Autodesk Fusion 360 part; units mm, degrees
(part 2 of 5)
sketch "Boceto1" plane through (0, 0, 0) normal (0, 1, 0) x (1, 0, 0)
  line L0 (4.8, 0) -> (4.8, -7)
  line L1 (4.8, -7) -> (0, -7)
  line L2 (0, -7) -> (0, 0)
  line L3 (49.6, 0) -> (49.6, -7)
  line L4 (49.6, -7) -> (44.8, -7)
  line L5 (44.8, -7) -> (44.8, 0)
  line L6 (0, 0) -> (-6, 0)
  line L7 (-6, 0) -> (-6, -10)
  line L8 (24.8, 0) -> (24.8, -18)
  line L9 (-2, -14) -> (24.8, -14)
  line L10 (4.8, 0) -> (44.8, 0)
  line L11 (51.6, -14) -> (24.8, -14)
  line L12 (55.6, 0) -> (55.6, -10)
  line L13 (49.6, 0) -> (55.6, 0)
  line L14 (-6, -10) -> (-2, -14)
  line L15 (51.6, -14) -> (55.6, -10)
  line L16 (17.8431, -4) -> (24.8, -11)
  line L17 (17.8431, -4) -> (24.8, -4)
  line L18 (9.8, -3) -> (16.7569, -10)
  line L19 (16.7569, -10) -> (9.8, -10)
  line L20 (9.8, -10) -> (9.8, -3)
  line L21 (39.8, -3) -> (32.8431, -10)
  line L22 (39.8, -10) -> (39.8, -3)
  line L23 (32.8431, -10) -> (39.8, -10)
  line L24 (31.7569, -4) -> (24.8, -4)
  line L25 (31.7569, -4) -> (24.8, -11)
  arc A0 (51.6, -14) -> (-2, -14) centre (24.8, -513.2812) ccw
  point P0 (-6, -14)
  point P1 (55.6, -14)
  dimension "d1" = 4.8
  dimension "d2" = 7
  dimension "d3" = 7
  dimension "d4" = 4.8
  dimension "d5" = 40
  dimension "d6" = 14
  dimension "d8" = 40
  dimension "d9" = 6
  dimension "d10" = 4
  dimension "d11" = 4
  dimension "d12" = 4
  dimension "d13" = 4
  dimension "d14" = 5
  dimension "d15" = 4
  dimension "d16" = 3
  dimension "d17" = 5
  dimension "d18" = 4
  dimension "d19" = 3
  dimension "d26" = 500
  constraint vertical L0
  constraint horizontal L1
  constraint vertical L2
  constraint coincident L2.end L6.start
  constraint vertical L3
  constraint horizontal L4
  constraint vertical L5
  constraint perpendicular L2 L6
  constraint perpendicular L6 L7
  constraint vertical L8
  constraint coincident L8 L9.end
  constraint perpendicular L8 L9
  constraint symmetric L2.end L8 L3.start
  constraint symmetric L6.end L8 L12.start
  constraint symmetric P0 L8 P1
  constraint symmetric L8 L9.end L11.end
  constraint coincident L8.start L10
  constraint coincident L5.end L6
  constraint horizontal L10
  constraint coincident P0 L7
  constraint coincident P0 L9
  constraint coincident P1 L11
  constraint coincident P1 L12
  constraint coincident L8 L16.end
  constraint coincident L8 L17.end
  constraint perpendicular L8 L17
  constraint parallel L17 L19
  constraint vertical L20
  constraint parallel L16 L18
  constraint symmetric L8 L16.start L24.start
  constraint symmetric L8 L16.end L25.end
  constraint symmetric L8 L17.end L24.end
  constraint symmetric L8 L18.start L21.start
  constraint symmetric L8 L18.end L21.end
  constraint symmetric L8 L19.end L22.start
  measures "d1" distance of L2.end L0.start
  measures "d2" distance of L2.end L1.end
  measures "d3" distance of L5.end L4.end
  measures "d4" distance of L5.end L3.start
  measures "d5" distance of L0 L5
  measures "d6" distance of L6.end P0
  measures "d9" distance of L2.end L6.end
  measures "d10" distance of P0 L7.end
  measures "d11" distance of P0 L9.start
  measures "d12" distance of P1 L11.start
  measures "d13" distance of P1 L12.end
  measures "d14" distance of L0 L20
  measures "d15" distance of L9 L19
  measures "d16" distance of L10 L18.start
  measures "d17" distance of L16 L18
  measures "d18" distance of L10 L17
  measures "d19" distance of L11 L16.end
  measures "d26" radius of A0
extrude "Extruir1" add sketch "Boceto1" along normal blind 4.8 contours L0 L1 L2 L6 L7 L8 L10 L14 L16 L17 A0 | L3 L4 L5 L8 L10 L12 L13 L15 L24 L25 A0
fillet "Empalme1" radius 1 9 edges at (9.8, 2.4, 3) (9.8, 2.4, 10) (16.7569, 2.4, 10) (17.8431, 2.4, 4) (24.8, 2.4, 11) (31.7569, 2.4, 4) (32.8431, 2.4, 10) (39.8, 2.4, 3) (39.8, 2.4, 10)
fillet "Empalme2" radius 2.5 4 edges at (-6, 2.4, 10) (55.6, 2.4, 10) (51.6, 2.4, 14) (-2, 2.4, 14)
sketch "Boceto2" plane through (0, 0, 0) normal (0, -1, 0) x (1, 0, 0)
  arc A0 (15.0624, 8.2951) -> (14.3532, 10) centre (14.3532, 9) ccw
  line L0 (15.0624, 8.2951) -> (11.5093, 4.7199)
  arc A1 (9.8, 5.4248) -> (11.5093, 4.7199) centre (10.8, 5.4248) ccw
  line L1 (9.8, 5.4248) -> (9.8, 9)
  arc A2 (10.8, 10) -> (9.8, 9) centre (10.8, 9) ccw
  line L2 (10.8, 10) -> (14.3532, 10)
  arc A3 (39.8, 9) -> (38.8, 10) centre (38.8, 9) ccw
  line L3 (39.8, 9) -> (39.8, 5.4248)
  arc A4 (38.0907, 4.7199) -> (39.8, 5.4248) centre (38.8, 5.4248) ccw
  line L4 (38.0907, 4.7199) -> (34.5376, 8.2951)
  arc A5 (35.2468, 10) -> (34.5376, 8.2951) centre (35.2468, 9) ccw
  line L5 (35.2468, 10) -> (38.8, 10)
  arc A6 (25.5093, 10.2863) -> (24.0907, 10.2863) centre (24.8, 9.5814) ccw
  line L6 (25.5093, 10.2863) -> (30.0624, 5.7049)
  arc A7 (29.3532, 4) -> (30.0624, 5.7049) centre (29.3532, 5) ccw
  line L7 (29.3532, 4) -> (20.2468, 4)
  arc A8 (19.5376, 5.7049) -> (20.2468, 4) centre (20.2468, 5) ccw
  line L8 (19.5376, 5.7049) -> (24.0907, 10.2863)
  arc A9 (-0.891, 13.9417) -> (-2.7872, 13.2128) centre (-1.0195, 11.445) ccw
  line L9 (-2.7872, 13.2128) -> (-5.2678, 10.7322)
  arc A10 (-5.2678, 10.7322) -> (-6, 8.9645) centre (-3.5, 8.9645) ccw
  line L10 (-6, 8.9645) -> (-6, 0)
  line L11 (-6, 0) -> (0, 0)
  line L12 (0, 0) -> (0, 7)
  line L13 (0, 7) -> (4.8, 7)
  line L14 (4.8, 7) -> (4.8, 0)
  line L15 (4.8, 0) -> (44.8, 0)
  line L16 (44.8, 0) -> (44.8, 7)
  line L17 (44.8, 7) -> (49.6, 7)
  line L18 (49.6, 7) -> (49.6, 0)
  line L19 (49.6, 0) -> (55.6, 0)
  line L20 (55.6, 0) -> (55.6, 8.9645)
  arc A11 (55.6, 8.9645) -> (54.8678, 10.7322) centre (53.1, 8.9645) ccw
  line L21 (54.8678, 10.7322) -> (52.3872, 13.2128)
  arc A12 (52.3872, 13.2128) -> (50.491, 13.9417) centre (50.6195, 11.445) ccw
  arc A13 (-0.891, 13.9417) -> (50.491, 13.9417) centre (24.8, 513.2812) ccw
extrude "Extruir2" add 3 faces at (-2, 1.6, 0) (18.1333, 1.6, 0) (51.6, 1.6, 0) along direction (0, 0, -1) blind 2
chamfer "Chaflán1" distance 1 angle 45 4 edges at (0, 2.4, -2) (4.8, 2.4, -2) (44.8, 2.4, -2) (49.6, 2.4, -2)
sketch "Boceto3" plane through (0, 0, 0) normal (0, -1, 0) x (1, 0, 0)
  line L0 (49.6, -1) -> (50.6, -2)
  line L1 (50.6, -2) -> (55.6, -2)
  line L2 (55.6, -2) -> (55.6, 0)
  line L3 (55.6, 0) -> (55.6, 8.9645)
  arc A0 (55.6, 8.9645) -> (54.8678, 10.7322) centre (53.1, 8.9645) ccw
  line L4 (54.8678, 10.7322) -> (52.3872, 13.2128)
  arc A1 (52.3872, 13.2128) -> (50.491, 13.9417) centre (50.6195, 11.445) ccw
  arc A2 (-0.891, 13.9417) -> (50.491, 13.9417) centre (24.8, 513.2812) ccw
  arc A3 (-0.891, 13.9417) -> (-2.7872, 13.2128) centre (-1.0195, 11.445) ccw
  line L5 (-2.7872, 13.2128) -> (-5.2678, 10.7322)
  arc A4 (-5.2678, 10.7322) -> (-6, 8.9645) centre (-3.5, 8.9645) ccw
  line L6 (-6, 8.9645) -> (-6, -2)
  line L7 (-6, -2) -> (-1, -2)
  line L8 (-1, -2) -> (0, -1)
  line L9 (0, -1) -> (0, 7)
  line L10 (0, 7) -> (4.8, 7)
  line L11 (4.8, 7) -> (4.8, -1)
  line L12 (4.8, -1) -> (5.8, -2)
  line L13 (5.8, -2) -> (43.8, -2)
  line L14 (43.8, -2) -> (44.8, -1)
  line L15 (44.8, -1) -> (44.8, 7)
  line L16 (44.8, 7) -> (49.6, 7)
  line L17 (49.6, 7) -> (49.6, -1)
  arc A5 (15.0624, 8.2951) -> (14.3532, 10) centre (14.3532, 9) ccw
  line L18 (15.0624, 8.2951) -> (11.5093, 4.7199)
  arc A6 (9.8, 5.4248) -> (11.5093, 4.7199) centre (10.8, 5.4248) ccw
  line L19 (9.8, 5.4248) -> (9.8, 9)
  arc A7 (10.8, 10) -> (9.8, 9) centre (10.8, 9) ccw
  line L20 (10.8, 10) -> (14.3532, 10)
  arc A8 (39.8, 9) -> (38.8, 10) centre (38.8, 9) ccw
  line L21 (39.8, 9) -> (39.8, 5.4248)
  arc A9 (38.0907, 4.7199) -> (39.8, 5.4248) centre (38.8, 5.4248) ccw
  line L22 (38.0907, 4.7199) -> (34.5376, 8.2951)
  arc A10 (35.2468, 10) -> (34.5376, 8.2951) centre (35.2468, 9) ccw
  line L23 (35.2468, 10) -> (38.8, 10)
  arc A11 (25.5093, 10.2863) -> (24.0907, 10.2863) centre (24.8, 9.5814) ccw
  line L24 (25.5093, 10.2863) -> (30.0624, 5.7049)
  arc A12 (29.3532, 4) -> (30.0624, 5.7049) centre (29.3532, 5) ccw
  line L25 (29.3532, 4) -> (20.2468, 4)
  arc A13 (19.5376, 5.7049) -> (20.2468, 4) centre (20.2468, 5) ccw
  line L26 (19.5376, 5.7049) -> (24.0907, 10.2863)
equation "d3 = d2"
equation "d4 = d1"
equation "d6 = d2 * 2"
equation "d8 = d5"
equation "d11 = d10"
equation "d13 = d12"
equation "d18 = d15"
equation "d19 = d16"

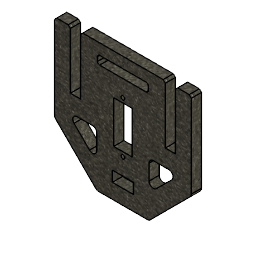
design "SOPORTE SERVO"
Autodesk Fusion 360 part; units mm, degrees
sketch "Boceto1" plane through (0, 0, 0) normal (0, 1, 0) x (1, 0, 0)
  line L0 (0, -1.75) -> (0, -22.5)
  line L1 (-32.3, 1.3953) -> (-32.3, 26)
  line L2 (-32.3, 27.5) -> (47.5, 27.5) construction
  circle A0 centre (0, 27.5) radius 10 construction
  line L3 (-4.35, 39) -> (4.35, 39)
  line L4 (4.35, 39) -> (4.35, 19.1)
  line L5 (4.35, 19.1) -> (-4.35, 19.1)
  line L6 (-4.35, 19.1) -> (-4.35, 39)
  line L7 (-28.6363, 33.7364) -> (-12.7638, 46.7364)
  line L8 (-6.4275, 49) -> (6.4275, 49)
  line L9 (-24.8, -0.2999) -> (-24.8, 27.5)
  line L10 (-24.8, 27.5) -> (-20, 27.5)
  line L11 (-20, 27.5) -> (-20, 0.025)
  line L12 (20, 27.5) -> (20, 0.025)
  line L13 (24.8, -0.2999) -> (24.8, 27.5)
  line L14 (24.8, 27.5) -> (20, 27.5)
  arc A1 (-25.2684, -0.7989) -> (-29.6149, -1.0978) centre (0, -400) ccw
  arc A2 (20, -0.5003) -> (24.8, -0.7695) centre (0, -400) ccw construction
  arc A3 (29.6164, -1.0979) -> (25.2684, -0.7989) centre (0, -400) ccw
  arc A4 (19.4757, -0.4744) -> (-19.4757, -0.4744) centre (0, -400) ccw
  arc A5 (-32.3, 1.3953) -> (-29.6149, -1.0978) centre (-29.8, 1.3953) ccw
  arc A6 (-28.6363, 33.7364) -> (-32.3, 26) centre (-22.3, 26) ccw
  arc A7 (-6.4275, 49) -> (-12.7638, 46.7364) centre (-6.4275, 39) ccw
  arc A8 (29.6149, -1.0978) -> (32.3, 1.3953) centre (29.8, 1.3953) ccw
  line L15 (32.3, 1.3953) -> (32.3, 26)
  arc A9 (32.3, 26) -> (28.6363, 33.7364) centre (22.3, 26) ccw
  line L16 (28.6363, 33.7364) -> (12.7638, 46.7364)
  arc A10 (12.7638, 46.7364) -> (6.4275, 49) centre (6.4275, 39) ccw
  line L17 (20, 27.5) -> (24.8, 27.5)
  circle A11 centre (0, 17) radius 0.9
  line L18 (4.35, 29.05) -> (-4.35, 29.05)
  circle A12 centre (0, 41.1) radius 0.9
  arc A13 (-25.2684, -0.7989) -> (-24.8, -0.2999) centre (-25.3, -0.2999) ccw
  arc A14 (-20, 0.025) -> (-19.4757, -0.4744) centre (-19.5, 0.025) ccw
  arc A15 (19.4757, -0.4744) -> (20, 0.025) centre (19.5, 0.025) ccw
  arc A16 (24.8, -0.2999) -> (25.2684, -0.7989) centre (25.3, -0.2999) ccw
  line L19 (-13, 5) -> (-13, 35.1269)
  line L20 (-11.1681, 38.9951) -> (-11.0225, 39.1144)
  line L21 (-9.39, 38.2925) -> (-11.0012, 4.9517)
  arc A17 (-13, 5) -> (-11.0012, 4.9517) centre (-12, 5) ccw
  arc A18 (-9.39, 38.2925) -> (-11.0225, 39.1144) centre (-10.3889, 38.3407) ccw
  arc A19 (-11.1681, 38.9951) -> (-13, 35.1269) centre (-8, 35.1269) ccw
  arc A20 (13, 35.1269) -> (11.1681, 38.9951) centre (8, 35.1269) ccw
  line L22 (11.1681, 38.9951) -> (11.0225, 39.1144)
  line L23 (9.39, 38.2925) -> (11.0012, 4.9517)
  line L24 (13, 5) -> (13, 35.1269)
  arc A21 (11.0012, 4.9517) -> (13, 5) centre (12, 5) ccw
  arc A22 (11.0225, 39.1144) -> (9.39, 38.2925) centre (10.3889, 38.3407) ccw
  arc A23 (2.8978, 9.7765) -> (0, 6) centre (0, 9) ccw
  line L25 (7.6073, -0.0723) -> (4.8296, 10.2941)
  arc A24 (4.8296, 10.2941) -> (0, 4) centre (0, 9) ccw
  line L26 (2.8978, 9.7765) -> (5.5276, -0.0382)
  arc A25 (0, 4) -> (0, 6) centre (0, 5) ccw
  point P0 (-35.0297, 28.5)
  point P1 (-10, 49)
  point P2 (10, 49)
  point P3 (0, 41.1)
  point P4 (10.3889, 38.3407)
  dimension "d1" = 800
  dimension "d2" = 20
  dimension "d3" = 8.7
  dimension "d4" = 19.9
  dimension "d5" = 4.35
  dimension "d6" = 8.4
  dimension "d7" = 27.5
  dimension "d10" = 20
  dimension "d11" = 10
  dimension "d12" = 10
  dimension "d13" = 4.8
  dimension "d14" = 7.5
  dimension "d15" = 1
  dimension "d17" = 2.5
  dimension "d18" = 10
  dimension "d19" = 1.5
  dimension "d20" = 1.8
  dimension "d21" = 2.1
  dimension "d22" = 0.5
  dimension "d23" = 0.5
  dimension "d24" = 7
  dimension "d25" = 7
  dimension "d30" = 5
  dimension "d32" = 1
  dimension "d33" = 5
  dimension "d36" = 40
  dimension "d37" = 20
  dimension "d38" = 2
  dimension "d39" = 5
  dimension "d41" = 3
  dimension "d42" = 15
  dimension "d43" = 5
  dimension "d44" = 2
  constraint coincident origin A2
  constraint coincident A1.centre L0
  constraint vertical L1
  constraint perpendicular L1 L2
  constraint coincident L0 A0.centre
  constraint horizontal L3
  constraint vertical L4
  constraint horizontal L5
  constraint vertical L6
  constraint coincident L2 A0.centre
  constraint perpendicular L1 L8
  constraint coincident L2 L9.end
  constraint perpendicular L2 L9
  constraint equal A2 A3
  constraint coincident L2 L10.end
  constraint vertical L11
  constraint coincident L1 L2.start
  constraint symmetric L0 L9.end L13.end
  constraint symmetric L0 L10.end L12.start
  constraint concentric A1 A4
  constraint concentric A3 A4
  constraint tangent L1 A5
  constraint tangent A1 A5
  constraint coincident P0 L7
  constraint tangent L1 A6
  constraint tangent L7 A6
  constraint coincident P1 L7
  constraint coincident P1 L8
  constraint tangent L7 A7
  constraint tangent L8 A7
  constraint equal A6 A7
  constraint coincident P2 L8
  constraint symmetric L0 L1.start A8.end
  constraint symmetric L0 A1.end A8.start
  constraint symmetric L0 A5 A8
  constraint symmetric L0 L1.end L15.end
  constraint symmetric L0 L7.start A9.end
  constraint symmetric L0 A6 A9
  constraint symmetric L0 L7.end L16.end
  constraint symmetric L0 L8.start L8.end
  constraint symmetric L0 A7 A10
  constraint coincident A3.start A8
  constraint coincident L0 A11.centre
  constraint midpoint L4 L18.start
  constraint midpoint L6 L18.end
  constraint symmetric A11.centre L18 P3
  constraint symmetric A11 L18 A12
  constraint tangent L9 A13
  constraint tangent A1 A13
  constraint tangent L11 A14
  constraint tangent A4 A14
  constraint equal A13 A14
  constraint coincident A2.start L12
  constraint coincident A2.start A4
  constraint tangent A4 A15
  constraint tangent L12 A15
  constraint equal A13 A15
  constraint coincident A2.end L13
  constraint coincident A2.end A3
  constraint tangent A3 A16
  constraint tangent L13 A16
  constraint equal A1 A2
  constraint equal A2 A4
  constraint vertical L12
  constraint vertical L13
  constraint perpendicular L2 L19
  constraint parallel L7 L20
  constraint tangent L19 A17
  constraint tangent L21 A17
  constraint tangent L21 A18
  constraint tangent L20 A18
  constraint equal A17 A18
  constraint tangent L19 A19
  constraint tangent L20 A19
  constraint symmetric L0 L19.start L24.start
  constraint symmetric L0 L21.end L23.end
  constraint symmetric L0 A17 A21
  constraint symmetric L0 L21.start L23.start
  constraint symmetric L0 L20.end L22.end
  constraint symmetric L0 A18.centre P4
  constraint symmetric L0 L19.end A20.start
  constraint symmetric L0 L20.start A20.end
  constraint symmetric L0 A19 A20
  constraint symmetric L0 A18 A22
  constraint tangent A23 A25
  constraint coincident L0 A25.centre
  constraint coincident L0 A23.centre
  constraint concentric A23 A24
  constraint coincident A2 L25.start
  constraint coincident A2 L26.end
  constraint tangent A23 L26
  constraint parallel L25 L26
  constraint tangent L25 A24
  measures "d1" diameter of A2
  measures "d2" diameter of A0
  measures "d3" distance of L3.start L3.end
  measures "d4" distance of L3.start L5.end
  measures "d5" distance of origin L6
  measures "d6" distance of A0.centre L5
  measures "d7" distance of origin L2
  measures "d10" distance of P1 P2
  measures "d11" distance of L3 L8
  measures "d12" horizontal distance of A0.centre P1
  measures "d13" distance of L9.end L10.end
  measures "d14" distance of L1 L9
  measures "d15" distance of P0 L2
  measures "d17" radius of A5
  measures "d18" radius of A6
  measures "d19" distance of L2 A6.centre
  measures "d20" diameter of A11
  measures "d21" distance of L5 A11.centre
  measures "d22" radius of A13
  measures "d23" radius of A16
  measures "d24" distance of L7 L20
  measures "d25" distance of L11 L19
  measures "d30" distance of L3.start L21
  measures "d32" radius of A17
  measures "d33" radius of A19
  measures "d36" distance of L11 L12
  measures "d37" distance of A0.centre L11
  measures "d38" diameter of A25
  measures "d39" distance of origin A25.centre
  measures "d41" radius of A23
  measures "d42" angle of L0 L26
  measures "d43" vertical distance of origin A17.centre
  measures "d44" distance of A23 A24
extrude "Extruir1" add sketch "Boceto1" along normal blind 4.8 contours L1 L7 L8 L9 L10 L11 L12 L13 L14 A1 A3 A4 A5 A6 A7 A8 L15 A9 L16 A10 L17 A13 A14 A15 A16 A23 L25 A24 L26 A25
sketch "Boceto3" plane through (0, 0, 0) normal (0, -1, 0) x (1, 0, 0)
  arc A0 (9.39, -38.2925) -> (11.0225, -39.1144) centre (10.3889, -38.3407) ccw
  line L0 (9.39, -38.2925) -> (11.0012, -4.9517)
  arc A1 (13, -5) -> (11.0012, -4.9517) centre (12, -5) ccw
  line L1 (13, -5) -> (13, -35.1269)
  arc A2 (11.1681, -38.9951) -> (13, -35.1269) centre (8, -35.1269) ccw
  line L2 (11.1681, -38.9951) -> (11.0225, -39.1144)
  arc A3 (-11.0225, -39.1144) -> (-9.39, -38.2925) centre (-10.3889, -38.3407) ccw
  line L3 (-11.0225, -39.1144) -> (-11.1681, -38.9951)
  arc A4 (-13, -35.1269) -> (-11.1681, -38.9951) centre (-8, -35.1269) ccw
  line L4 (-13, -35.1269) -> (-13, -5)
  arc A5 (-11.0012, -4.9517) -> (-13, -5) centre (-12, -5) ccw
  line L5 (-11.0012, -4.9517) -> (-9.39, -38.2925)
  line L6 (-4.35, -19.1) -> (4.35, -19.1)
  line L7 (4.35, -19.1) -> (4.35, -39)
  line L8 (4.35, -39) -> (-4.35, -39)
  line L9 (-4.35, -39) -> (-4.35, -19.1)
  circle A6 centre (0, -17) radius 0.9
  circle A7 centre (0, -41.1) radius 0.9
  arc A8 (20, -0.025) -> (19.4757, 0.4744) centre (19.5, -0.025) ccw
  arc A9 (7.6073, 0.0723) -> (19.4757, 0.4744) centre (0, 400) ccw
  line L10 (7.6073, 0.0723) -> (4.8296, -10.2941)
  arc A10 (0, -4) -> (4.8296, -10.2941) centre (0, -9) ccw
  arc A11 (0, -6) -> (0, -4) centre (0, -5) ccw
  arc A12 (0, -6) -> (2.8978, -9.7765) centre (0, -9) ccw
  line L11 (2.8978, -9.7765) -> (5.5276, 0.0382)
  arc A13 (-19.4757, 0.4744) -> (5.5276, 0.0382) centre (0, 400) ccw
  arc A14 (-19.4757, 0.4744) -> (-20, -0.025) centre (-19.5, -0.025) ccw
  line L12 (-20, -0.025) -> (-20, -27.5)
  line L13 (-20, -27.5) -> (-24.8, -27.5)
  line L14 (-24.8, -27.5) -> (-24.8, 0.2999)
  arc A15 (-24.8, 0.2999) -> (-25.2684, 0.7989) centre (-25.3, 0.2999) ccw
  arc A16 (-29.6149, 1.0978) -> (-25.2684, 0.7989) centre (0, 400) ccw
  arc A17 (-29.6149, 1.0978) -> (-32.3, -1.3953) centre (-29.8, -1.3953) ccw
  line L15 (-32.3, -1.3953) -> (-32.3, -26)
  arc A18 (-32.3, -26) -> (-28.6363, -33.7364) centre (-22.3, -26) ccw
  line L16 (-28.6363, -33.7364) -> (-12.7638, -46.7364)
  arc A19 (-12.7638, -46.7364) -> (-6.4275, -49) centre (-6.4275, -39) ccw
  line L17 (-6.4275, -49) -> (6.4275, -49)
  arc A20 (6.4275, -49) -> (12.7638, -46.7364) centre (6.4275, -39) ccw
  line L18 (12.7638, -46.7364) -> (28.6363, -33.7364)
  arc A21 (28.6363, -33.7364) -> (32.3, -26) centre (22.3, -26) ccw
  line L19 (32.3, -26) -> (32.3, -1.3953)
  arc A22 (32.3, -1.3953) -> (29.6149, 1.0978) centre (29.8, -1.3953) ccw
  arc A23 (25.2684, 0.7989) -> (29.6149, 1.0978) centre (0, 400) ccw
  arc A24 (25.2684, 0.7989) -> (24.8, 0.2999) centre (25.3, 0.2999) ccw
  line L20 (24.8, 0.2999) -> (24.8, -27.5)
  line L21 (24.8, -27.5) -> (20, -27.5)
  line L22 (20, -27.5) -> (20, -0.025)
  line L23 (-5, -49) -> (5, -49)
  line L24 (5, -49) -> (5, -54)
  line L25 (5, -54) -> (-5, -54)
  line L26 (-5, -54) -> (-5, -49)
  line L27 (-12.3, -61) -> (12.3, -61)
  line L28 (32.3, -41) -> (32.3, -26)
  line L29 (-32.3, -41) -> (-32.3, -26)
  line L30 (12.3, -61) -> (32.3, -41)
  line L31 (-12.3, -61) -> (-32.3, -41)
  arc A25 (-19.4757, 0.4744) -> (19.4757, 0.4744) centre (0, 400) ccw
  line L32 (-20, -0.025) -> (-20, 0.5003)
  line L33 (20, -0.025) -> (20, 0.5003)
  arc A26 (-20, 0.5003) -> (-19.4757, 0.4744) centre (0, 400) ccw
  arc A27 (19.4757, 0.4744) -> (20, 0.5003) centre (0, 400) ccw
  point P0 (-32.3, -61)
  point P1 (32.3, -61)
  dimension "d45" = 5
  dimension "d46" = 5
  dimension "d47" = 10
  dimension "d48" = 7
  dimension "d49" = 20
  dimension "d50" = 20
  dimension "d51" = 20
  dimension "d52" = 20
  constraint horizontal L23
  constraint vertical L24
  constraint horizontal L25
  constraint vertical L26
  constraint coincident L17 L23.start
  constraint perpendicular L26 L27
  constraint coincident A21.end L19.start
  constraint vertical L28
  constraint coincident L15.end A18.start
  constraint vertical L29
  constraint coincident P1 L27
  constraint coincident P1 L28
  constraint coincident P0 L27
  constraint coincident P0 L29
  constraint tangent A9 A25
  constraint tangent A8 A25
  constraint coincident A13.start A14.start
  constraint coincident A14.end L12.start
  constraint vertical L32
  constraint coincident A25 L32.end
  constraint coincident A8.start L22.end
  constraint tangent A8 L33
  constraint equal A25 A26
  constraint coincident A8 A9.end
  constraint coincident A25 L33.end
  constraint coincident L33.end A27.end
  constraint coincident A9.centre A13.centre
  measures "d45" distance of L23.start L25.end
  measures "d46" distance of A7.centre L24
  measures "d47" distance of L24 L26
  measures "d48" distance of L25 L27
  measures "d49" distance of P1 L27.end
  measures "d50" distance of P1 L28.start
  measures "d51" distance of P0 L27.start
  measures "d52" distance of P0 L29.start
extrude "Extruir2" add sketch "Boceto3" against normal blind 4.8 contours A0 L0 A1 L1 A2 L2 | A3 L3 A4 L4 A5 L5 | A8 L33 A27 | L10 A10 A11 A12 L11 A25 | A14 L32 A26 | A18 L16 A19 L17 A20 L18 A21 L24 L25 L26 L27 L28 L29 L30 L31
sketch "Boceto4" plane through (0, 0, 0) normal (0, -1, 0) x (1, 0, 0)
  line L0 (32.3, -41) -> (32.3, -1.3953)
  arc A0 (32.3, -1.3953) -> (29.6149, 1.0978) centre (29.8, -1.3953) ccw
  arc A1 (25.2684, 0.7989) -> (29.6149, 1.0978) centre (0, 400) ccw
  arc A2 (25.2684, 0.7989) -> (24.8, 0.2999) centre (25.3, 0.2999) ccw
  line L1 (24.8, 0.2999) -> (24.8, -27.5)
  line L2 (24.8, -27.5) -> (20, -27.5)
  line L3 (20, -27.5) -> (20, 0.5003)
  arc A3 (-19.4757, 0.4744) -> (20, 0.5003) centre (0, 400) ccw
  line L4 (-20, 0.5003) -> (-20, -27.5)
  line L5 (-20, -27.5) -> (-24.8, -27.5)
  line L6 (-24.8, -27.5) -> (-24.8, 0.2999)
  arc A4 (-24.8, 0.2999) -> (-25.2684, 0.7989) centre (-25.3, 0.2999) ccw
  arc A5 (-29.6149, 1.0978) -> (-25.2684, 0.7989) centre (0, 400) ccw
  arc A6 (-29.6149, 1.0978) -> (-32.3, -1.3953) centre (-29.8, -1.3953) ccw
  line L7 (-32.3, -1.3953) -> (-32.3, -41)
  line L8 (-32.3, -41) -> (-12.3, -61)
  line L9 (-12.3, -61) -> (12.3, -61)
  line L10 (12.3, -61) -> (32.3, -41)
  line L11 (-4.35, -19.1) -> (4.35, -19.1)
  line L12 (4.35, -19.1) -> (4.35, -39)
  line L13 (4.35, -39) -> (-4.35, -39)
  line L14 (-4.35, -39) -> (-4.35, -19.1)
  circle A7 centre (0, -17) radius 0.9
  circle A8 centre (0, -41.1) radius 0.9
  line L15 (5, -49) -> (5, -54)
  line L16 (5, -54) -> (-5, -54)
  line L17 (-5, -54) -> (-5, -49)
  line L18 (-5, -49) -> (5, -49)
  line L19 (-32.3, -7.5) -> (-24.8, -7.5)
  line L20 (24.8, -7.5) -> (32.3, -7.5)
  line L21 (-24.3, -37.6863) -> (-12.35, -49.6363)
  line L22 (-12.35, -49.6363) -> (-12.35, -37.6863)
  line L23 (-24.3, -37.6863) -> (-24.3, -35.5)
  line L24 (-24.3, -35.5) -> (-12.35, -35.5)
  line L25 (-12.35, -35.5) -> (-12.35, -37.6863)
  line L26 (0, 1.75) -> (0, 22.5)
  line L27 (24.3, -37.6863) -> (12.35, -49.6363)
  line L28 (24.3, -37.6863) -> (24.3, -35.5)
  line L29 (24.3, -35.5) -> (12.35, -35.5)
  line L30 (12.35, -49.6363) -> (12.35, -37.6863)
  line L31 (12.35, -35.5) -> (12.35, -37.6863)
  arc A9 (-20, 0.5003) -> (-19.4757, 0.4744) centre (0, 400) ccw
  dimension "d55" = 20
  dimension "d56" = 8
  dimension "d57" = 8
  dimension "d58" = 8
  dimension "d59" = 8
  constraint coincident L7 L19.start
  constraint coincident L6 L19.end
  constraint perpendicular L6 L19
  constraint coincident L1 L20.start
  constraint coincident L0 L20.end
  constraint perpendicular L0 L20
  constraint coincident L19 L20.start
  constraint vertical L22
  constraint parallel L8 L21
  constraint perpendicular L23 L24
  constraint vertical L25
  constraint symmetric L21.start L26 L27.start
  constraint symmetric L21.end L26 L27.end
  constraint symmetric L22.end L26 L30.end
  constraint symmetric L23.end L26 L28.end
  constraint symmetric L24.end L26 L29.end
  measures "d55" distance of L5 L19
  measures "d56" distance of L7 L21.start
  measures "d57" distance of L8 L21
  measures "d58" distance of L14 L22
  measures "d59" distance of L5 L24
extrude "Extruir3" cut sketch "Boceto4" against normal blind 4.8 contours L21 L22 L23 L24 L25 | L27 L28 L29 L30 L31
sketch "Boceto5" plane through (0, 0, 0) normal (0, -1, 0) x (1, 0, 0)
  line L0 (-32.3, -1.3953) -> (-32.3, -41)
  line L1 (-32.3, -41) -> (-12.3, -61)
  line L2 (-12.3, -61) -> (12.3, -61)
  line L3 (12.3, -61) -> (32.3, -41)
  line L4 (32.3, -41) -> (32.3, -1.3953)
  line L5 (24.8, 0.2999) -> (24.8, -27.5)
  line L6 (24.8, -27.5) -> (20, -27.5)
  line L7 (20, -27.5) -> (20, 0.5003)
  arc A0 (-19.4757, 0.4744) -> (20, 0.5003) centre (0, 400) ccw
  line L8 (-20, 0.5003) -> (-20, -27.5)
  line L9 (-20, -27.5) -> (-24.8, -27.5)
  line L10 (-24.8, -27.5) -> (-24.8, 0.2999)
  line L11 (5, -49) -> (5, -54)
  line L12 (5, -54) -> (-5, -54)
  line L13 (-5, -54) -> (-5, -49)
  line L14 (-5, -49) -> (5, -49)
  circle A1 centre (0, -41.1) radius 0.9
  circle A2 centre (0, -17) radius 0.9
  line L15 (-4.35, -19.1) -> (4.35, -19.1)
  line L16 (4.35, -19.1) -> (4.35, -39)
  line L17 (4.35, -39) -> (-4.35, -39)
  line L18 (-4.35, -39) -> (-4.35, -19.1)
  line L19 (12.35, -35.5) -> (24.3, -35.5)
  line L20 (24.3, -35.5) -> (24.3, -37.6863)
  line L21 (24.3, -37.6863) -> (12.35, -49.6363)
  line L22 (12.35, -49.6363) -> (12.35, -35.5)
  line L23 (-12.35, -35.5) -> (-12.35, -49.6363)
  line L24 (-12.35, -49.6363) -> (-24.3, -37.6863)
  line L25 (-24.3, -37.6863) -> (-24.3, -35.5)
  line L26 (-24.3, -35.5) -> (-12.35, -35.5)
  line L27 (-12, -9.1) -> (12, -9.1)
  line L28 (12, -9.1) -> (12, -5.1)
  line L29 (12, -5.1) -> (-12, -5.1)
  line L30 (-12, -5.1) -> (-12, -9.1)
  arc A3 (-24.8, 0.2999) -> (-25.2684, 0.7989) centre (-25.3, 0.2999) ccw
  arc A4 (-29.6149, 1.0978) -> (-25.2684, 0.7989) centre (0, 400) ccw
  arc A5 (-29.6149, 1.0978) -> (-32.3, -1.3953) centre (-29.8, -1.3953) ccw
  arc A6 (32.3, -1.3953) -> (29.6149, 1.0978) centre (29.8, -1.3953) ccw
  arc A7 (25.2684, 0.7989) -> (29.6149, 1.0978) centre (0, 400) ccw
  arc A8 (25.2684, 0.7989) -> (24.8, 0.2999) centre (25.3, 0.2999) ccw
  arc A9 (-20, 0.5003) -> (-19.4757, 0.4744) centre (0, 400) ccw
  dimension "d64" = 10
  dimension "d65" = 8
  dimension "d66" = 8
  dimension "d67" = 4
  constraint horizontal L27
  constraint vertical L28
  constraint horizontal L29
  constraint vertical L30
  measures "d64" distance of L15 L27
  measures "d65" distance of L8 L30
  measures "d66" distance of L7 L28
  measures "d67" distance of L27.end L28.end
extrude "Extruir4" cut sketch "Boceto5" against normal blind 4.8 contours L27 L28 L29 L30
fillet "Empalme2" radius 1 4 edges at (12, 2.4, -5.1) (12, 2.4, -9.1) (-12, 2.4, -9.1) (-12, 2.4, -5.1)
sketch "Boceto6" plane through (0, 0, 0) normal (0, -1, 0) x (1, 0, 0)
  line L0 (11, -9.1) -> (-11, -9.1)
  arc A0 (-12, -8.1) -> (-11, -9.1) centre (-11, -8.1) ccw
  line L1 (-12, -8.1) -> (-12, -6.1)
  arc A1 (-11, -5.1) -> (-12, -6.1) centre (-11, -6.1) ccw
  line L2 (-11, -5.1) -> (11, -5.1)
  arc A2 (12, -6.1) -> (11, -5.1) centre (11, -6.1) ccw
  line L3 (12, -6.1) -> (12, -8.1)
  arc A3 (11, -9.1) -> (12, -8.1) centre (11, -8.1) ccw
  line L4 (-12.35, -35.5) -> (-12.35, -49.6363)
  line L5 (-12.35, -49.6363) -> (-24.3, -37.6863)
  line L6 (-24.3, -37.6863) -> (-24.3, -35.5)
  line L7 (-24.3, -35.5) -> (-12.35, -35.5)
  line L8 (12.35, -35.5) -> (24.3, -35.5)
  line L9 (24.3, -35.5) -> (24.3, -37.6863)
  line L10 (24.3, -37.6863) -> (12.35, -49.6363)
  line L11 (12.35, -49.6363) -> (12.35, -35.5)
  line L12 (32.3, -41) -> (32.3, -1.3953)
  arc A4 (32.3, -1.3953) -> (29.6149, 1.0978) centre (29.8, -1.3953) ccw
  arc A5 (25.2684, 0.7989) -> (29.6149, 1.0978) centre (0, 400) ccw
  arc A6 (25.2684, 0.7989) -> (24.8, 0.2999) centre (25.3, 0.2999) ccw
  line L13 (24.8, 0.2999) -> (24.8, -27.5)
  line L14 (24.8, -27.5) -> (20, -27.5)
  line L15 (20, -27.5) -> (20, 0.5003)
  arc A7 (-19.4757, 0.4744) -> (20, 0.5003) centre (0, 400) ccw
  line L16 (-20, 0.5003) -> (-20, -27.5)
  line L17 (-20, -27.5) -> (-24.8, -27.5)
  line L18 (-24.8, -27.5) -> (-24.8, 0.2999)
  arc A8 (-24.8, 0.2999) -> (-25.2684, 0.7989) centre (-25.3, 0.2999) ccw
  arc A9 (-29.6149, 1.0978) -> (-25.2684, 0.7989) centre (0, 400) ccw
  arc A10 (-29.6149, 1.0978) -> (-32.3, -1.3953) centre (-29.8, -1.3953) ccw
  line L19 (-32.3, -1.3953) -> (-32.3, -41)
  line L20 (-32.3, -41) -> (-12.3, -61)
  line L21 (-12.3, -61) -> (12.3, -61)
  line L22 (12.3, -61) -> (32.3, -41)
  line L23 (-4.35, -19.1) -> (4.35, -19.1)
  line L24 (4.35, -19.1) -> (4.35, -39)
  line L25 (4.35, -39) -> (-4.35, -39)
  line L26 (-4.35, -39) -> (-4.35, -19.1)
  circle A11 centre (0, -17) radius 0.9
  circle A12 centre (0, -41.1) radius 0.9
  line L27 (5, -49) -> (5, -54)
  line L28 (5, -54) -> (-5, -54)
  line L29 (-5, -54) -> (-5, -49)
  line L30 (-5, -49) -> (5, -49)
  line L31 (-32.3, -10.188) -> (-32.3, 0)
  line L32 (-32.3, 0) -> (32.3, 0)
  line L33 (32.3, 0) -> (32.3, -10.3093)
  arc A13 (-20, 0.5003) -> (-19.4757, 0.4744) centre (0, 400) ccw
  dimension "d74" = 27.5
  constraint coincident L19 L31.start
  constraint perpendicular L31 L32
  constraint coincident L12 L33.end
  constraint horizontal L32
  constraint vertical L33
  measures "d74" distance of L14 L32
extrude "Extruir5" cut sketch "Boceto6" against normal blind 4.8 contours A4 A5 A6 L13 L32 | L15 A7 L32 | A7 L16 L32 A13 | L18 A8 A9 A10 L32
extrude "Extruir6" add sketch "Boceto6" against normal blind 4.8 contours A4 L32 L33 | A10 L31 L32
chamfer "Chaflán1" distance 1 angle 45 6 edges at (-32.3, 2.4, 0) (-24.8, 2.4, 0) (-20, 2.4, 0) (20, 2.4, 0) (24.8, 2.4, 0) (32.3, 2.4, 0)
fillet "Empalme4" radius 2 12 edges at (-32.3, 2.4, -41) (-12.35, 2.4, -35.5) (-24.3, 2.4, -35.5) (-24.3, 2.4, -37.6863) (-12.35, 2.4, -49.6363) (-12.3, 2.4, -61) (12.3, 2.4, -61) (12.35, 2.4, -49.6363) (12.35, 2.4, -35.5) (24.3, 2.4, -35.5) (24.3, 2.4, -37.6863) (32.3, 2.4, -41)
sketch "Boceto7" plane through (0, 0, 0) normal (0, -1, 0) x (1, 0, 0)
  line L0 (5, -49) -> (5, -54)
  line L1 (5, -54) -> (-5, -54)
  line L2 (-5, -54) -> (-5, -49)
  line L3 (-5, -49) -> (5, -49)
  circle A0 centre (0, -41.1) radius 0.9
  circle A1 centre (0, -17) radius 0.9
  line L4 (-4.35, -19.1) -> (4.35, -19.1)
  line L5 (4.35, -19.1) -> (4.35, -39)
  line L6 (4.35, -39) -> (-4.35, -39)
  line L7 (-4.35, -39) -> (-4.35, -19.1)
  line L8 (14.35, -35.5) -> (21.6579, -35.5)
  arc A2 (23.0721, -38.9142) -> (21.6579, -35.5) centre (21.6579, -37.5) ccw
  line L9 (23.0721, -38.9142) -> (15.7642, -46.2221)
  arc A3 (12.35, -44.8079) -> (15.7642, -46.2221) centre (14.35, -44.8079) ccw
  line L10 (12.35, -44.8079) -> (12.35, -37.5)
  arc A4 (14.35, -35.5) -> (12.35, -37.5) centre (14.35, -37.5) ccw
  arc A5 (-21.6579, -35.5) -> (-23.0721, -38.9142) centre (-21.6579, -37.5) ccw
  line L11 (-21.6579, -35.5) -> (-14.35, -35.5)
  arc A6 (-12.35, -37.5) -> (-14.35, -35.5) centre (-14.35, -37.5) ccw
  line L12 (-12.35, -37.5) -> (-12.35, -44.8079)
  arc A7 (-15.7642, -46.2221) -> (-12.35, -44.8079) centre (-14.35, -44.8079) ccw
  line L13 (-15.7642, -46.2221) -> (-23.0721, -38.9142)
  line L14 (11, -9.1) -> (-11, -9.1)
  arc A8 (-12, -8.1) -> (-11, -9.1) centre (-11, -8.1) ccw
  line L15 (-12, -8.1) -> (-12, -6.1)
  arc A9 (-11, -5.1) -> (-12, -6.1) centre (-11, -6.1) ccw
  line L16 (-11, -5.1) -> (11, -5.1)
  arc A10 (12, -6.1) -> (11, -5.1) centre (11, -6.1) ccw
  line L17 (12, -6.1) -> (12, -8.1)
  arc A11 (11, -9.1) -> (12, -8.1) centre (11, -8.1) ccw
  arc A12 (31.7142, -41.5858) -> (32.3, -40.1716) centre (30.3, -40.1716) ccw
  line L18 (32.3, -40.1716) -> (32.3, -1)
  line L19 (32.3, -1) -> (31.3, 0)
  line L20 (31.3, 0) -> (25.8, 0)
  line L21 (25.8, 0) -> (24.8, -1)
  line L22 (24.8, -1) -> (24.8, -27.5)
  line L23 (24.8, -27.5) -> (20, -27.5)
  line L24 (20, -27.5) -> (20, -1)
  line L25 (20, -1) -> (19, 0)
  line L26 (19, 0) -> (-19, 0)
  line L27 (-19, 0) -> (-20, -1)
  line L28 (-20, -1) -> (-20, -27.5)
  line L29 (-20, -27.5) -> (-24.8, -27.5)
  line L30 (-24.8, -27.5) -> (-24.8, -1)
  line L31 (-24.8, -1) -> (-25.8, 0)
  line L32 (-25.8, 0) -> (-31.3, 0)
  line L33 (-31.3, 0) -> (-32.3, -1)
  line L34 (-32.3, -1) -> (-32.3, -40.1716)
  arc A13 (-32.3, -40.1716) -> (-31.7142, -41.5858) centre (-30.3, -40.1716) ccw
  line L35 (-31.7142, -41.5858) -> (-12.8858, -60.4142)
  arc A14 (-12.8858, -60.4142) -> (-11.4716, -61) centre (-11.4716, -59) ccw
  line L36 (-11.4716, -61) -> (11.4716, -61)
  arc A15 (11.4716, -61) -> (12.8858, -60.4142) centre (11.4716, -59) ccw
  line L37 (12.8858, -60.4142) -> (31.7142, -41.5858)
equation "d5 = d3 / 2"
equation "d6 = 3.4 mm + 5 mm"
equation "d12 = d10 / 2"
equation "d37 = d36 / 2"
equation "d38 = d44"
equation "d47 = d46 * 2"
equation "d50 = d49"
equation "d52 = d51"

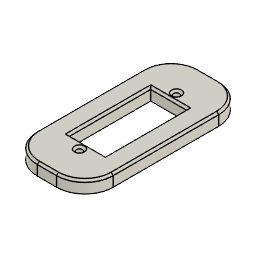
design "SOPORTE PLASTICO SERVO"
Autodesk Fusion 360 part; units mm, degrees
sketch "Boceto1" plane through (0, 0, 0) normal (0, 0, 1) x (1, 0, 0)
  line L0 (-4.3, -9.9) -> (4.3, -9.9) construction
  line L1 (4.3, -9.9) -> (4.3, 9.9) construction
  line L2 (4.3, 9.9) -> (-4.3, 9.9) construction
  line L3 (-4.3, 9.9) -> (-4.3, -9.9) construction
  line L4 (-4.3, -9.9) -> (4.3, 9.9) construction
  line L5 (4.3, -9.9) -> (-4.3, 9.9) construction
  line L6 (-4.45, -10.05) -> (4.45, -10.05)
  line L7 (4.45, -10.05) -> (4.45, 10.05)
  line L8 (4.45, 10.05) -> (-4.45, 10.05)
  line L9 (-4.45, 10.05) -> (-4.45, -10.05)
  line L10 (-2.375, -20.05) -> (2.375, -20.05)
  line L11 (9.375, -13.05) -> (9.375, 13.05)
  line L12 (2.375, 20.05) -> (-2.375, 20.05)
  line L13 (-9.375, 13.05) -> (-9.375, -13.05)
  arc A0 (-2.375, 20.05) -> (-9.375, 13.05) centre (-2.375, 13.05) ccw
  arc A1 (9.375, 13.05) -> (2.375, 20.05) centre (2.375, 13.05) ccw
  arc A2 (2.375, -20.05) -> (9.375, -13.05) centre (2.375, -13.05) ccw
  arc A3 (-9.375, -13.05) -> (-2.375, -20.05) centre (-2.375, -13.05) ccw
  circle A4 centre (0, 12) radius 0.75
  line L14 (0, 1.75) -> (0, 22.5)
  line L15 (1.75, 0) -> (22.5, 0)
  circle A5 centre (0, -12) radius 0.75
  dimension "d1" = 8.6
  dimension "d2" = 19.8
  dimension "d3" = 0.15
  dimension "d5" = 7
  dimension "d6" = 2.1
  dimension "d7" = 1.5
  dimension "d11" = 18.75
  dimension "d12" = 9.375
  constraint horizontal L0
  constraint perpendicular L0 L1
  constraint parallel L0 L2
  constraint parallel L1 L3
  constraint coincident L4 origin
  constraint coincident L5 origin
  constraint tangent L12 A0
  constraint tangent L13 A0
  constraint tangent L11 A1
  constraint tangent L12 A1
  constraint equal A0 A1
  constraint tangent L10 A2
  constraint tangent L11 A2
  constraint equal A0 A2
  constraint tangent L10 A3
  constraint tangent L13 A3
  constraint equal A0 A3
  constraint coincident A4.centre L14
  constraint symmetric A4 L15 A5
  constraint vertical L11
  measures "d1" distance of L1.end L2.end
  measures "d2" distance of L0.end L1.end
  measures "d5" radius of A0
  measures "d6" distance of L2 A4.centre
  measures "d7" diameter of A4
  measures "d11" distance of L11 L13
  measures "d12" distance of origin L13
extrude "Extruir1" add sketch "Boceto1" along normal blind 3 contours L6 L7 L8 L9 L10 L11 L12 L13 A0 A2 A3 A4 L14 L15 | L7 L8 L11 L12 A1 A4 L14 L15
chamfer "Chaflán1" distance 0.5 angle 45 1 faces at (-7.7333, 3.35, 3)
equation "d12 = d11 / 2"

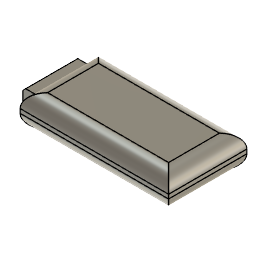
design "BATERIA"
Autodesk Fusion 360 part; units mm, degrees
sketch "Boceto1" plane through (0, 0, 0) normal (0, 0, 1) x (1, 0, 0)
  line L0 (0, 0) -> (54, 0)
  line L1 (54, 0) -> (54, 28.5)
  line L2 (54, 28.5) -> (0, 28.5)
  line L3 (0, 28.5) -> (0, 0)
  dimension "d1" = 54
  dimension "d2" = 28.5
  constraint horizontal L0
  constraint vertical L1
  constraint horizontal L2
  constraint vertical L3
  constraint coincident L0.start L3.end
  measures "d1" distance of L0.start L0.end
  measures "d2" distance of L0.start L2.end
extrude "Extruir1" add sketch "Boceto1" along normal blind 11.5
fillet "Empalme1" radius 5 2 faces at (18, 9.5, 11.5) (18, 9.5, 0)
sketch "Boceto2" plane through (0, 0, 0) normal (-1, 0, 0) x (0, -1, 0)
  line L0 (-28.5, 5) -> (0, 5)
  line L1 (0, 5) -> (0, 6.5)
  line L2 (0, 6.5) -> (-28.5, 6.5)
  line L3 (-28.5, 6.5) -> (-28.5, 5)
  line L4 (-25, 2.75) -> (-5, 2.75)
  line L5 (-5, 2.75) -> (-5, 8.75)
  line L6 (-5, 8.75) -> (-25, 8.75)
  line L7 (-25, 8.75) -> (-25, 2.75)
  dimension "d7" = 5
  dimension "d8" = 20
  dimension "d9" = 6
  dimension "d10" = 2.75
  constraint horizontal L4
  constraint vertical L5
  constraint horizontal L6
  constraint vertical L7
  measures "d7" distance of L1 L5
  measures "d8" distance of L4.start L4.end
  measures "d9" distance of L4.end L5.end
  measures "d10" distance of origin L4
extrude "Extruir2" add sketch "Boceto2" along normal blind 4 and the other way blind 1 contours L0 L2 L5 L7 | L0 L4 L5 L7 | L2 L5 L6 L7
chamfer "Chaflán1" distance 1 angle 45 5 edges at (-1.7326, 25, 8.75) (-1.7326, 25, 2.75) (-4, 15, 8.75) (-4, 15, 2.75) (-4, 25, 5.75)
equation "d10 = ( ( 11.5 - 6 ) / 2 ) * 1 mm"

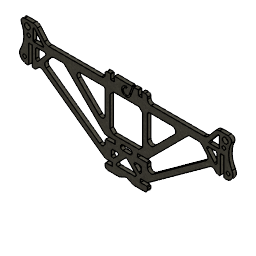
design "FRAME PRINCIPAL"
Autodesk Fusion 360 part; units mm, degrees